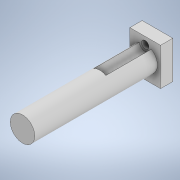
# Autodesk Inventor part: handle_vertical
Saved by Autodesk Inventor 2022.3 (Build 263350000, 350)
## iProperties
Created: 2022-06-10
Part Number: handle_vertical
Material: Generic
Document SubType Name: Modeling
Designer: Martijn
Density: 1 g/cm^3
Appearance: Default
Author: Martijn
Autodesk Inventor part; units mm, degrees
ref_plane "YZ Plane" through (0, 0, 0) normal (1, 0, 0) x (0, 1, 0)
ref_plane "XZ Plane" through (0, 0, 0) normal (0, 1, 0) x (-1, 0, 0)
ref_plane "XY Plane" through (0, 0, 0) normal (0, 0, 1) x (1, 0, 0)
sketch "Sketch1" plane through (0, 0, 0) normal (0, 0, 1) x (1, 0, 0)
  line L0 (0, 0) -> (25, 0)
  line L1 (25, 0) -> (25, 30.6)
  line L2 (25, 30.6) -> (0, 30.6)
  line L3 (0, 30.6) -> (0, 0)
  dimension "d0" = 25
  dimension "d1" = 30.6
  constraints: 8 end point, 2 parallel, 1 horizontal, 1 perpendicular
  measures "d0" distance of L0.start L0.end
  measures "d1" distance of L2.end L0.start
extrude "Extrusion1" add sketch "Sketch1" along normal blind 10
sketch "Sketch2" plane through (0, 0, 10) normal (0, 0, 1) x (1, 0, 0)
  circle A0 centre (12.5, 15.3) radius 10
  line L0 (25, 0) -> (25, 30.6) projected
  line L1 (0, 0) -> (25, 0) projected
  dimension "d4" = 12.5
  dimension "d6" = 20
  dimension "d19" = 15.3
  constraints: 1 centre point
  measures "d4" distance from line of L0 A0.centre
  measures "d6" diameter of A0
  measures "d19" distance from line of A0.centre L1
extrude "Extrusion2" add sketch "Sketch2" along normal blind 100
sketch "Sketch3" plane through (0, 0, 0) normal (0, 0, -1) x (-1, 0, 0)
  circle A0 centre (-12.5, 5.8) radius 3
  circle A1 centre (-12.5, 24.8) radius 3
  line L0 (0, 30.6) -> (0, 0) projected
  line L1 (0, 0) -> (-25, 0) projected
  point P0 (-12.5, 0)
  dimension "d9" = 6
  dimension "d10" = 6
  dimension "d11" = 12.5
  dimension "d12" = 12.5
  dimension "d13" = 19
  dimension "d14" = 5.8
  constraints: 2 centre point, 1 midpoint
  measures "d9" diameter of A0
  measures "d10" diameter of A1
  measures "d11" distance from line of L0 A0.centre
  measures "d12" distance from line of L0 A1.centre
  measures "d13" distance of A0.centre A1.centre
  measures "d14" distance of point (-12.5, 0) A0.centre
extrude "Extrusion3" cut sketch "Sketch3" against normal blind 20
sketch "Sketch4" plane through (0, 0, 10) normal (0, 0, 1) x (1, 0, 0)
  arc A0 (9.5003, 5.7605) -> (15.4997, 5.7605) centre (12.5, 5.8) ccw projected
  circle A1 centre (12.5, 5.8) radius 5
  arc A2 (15.4997, 24.8395) -> (9.5003, 24.8395) centre (12.5, 24.8) ccw projected
  circle A3 centre (12.5, 24.8) radius 5
  point P0 (0, 0)
  dimension "d17" = 10
  dimension "d18" = 10
  constraints: 2 centre point, 2 coincident
  measures "d17" diameter of A1
  measures "d18" diameter of A3
extrude "Extrusion4" cut sketch "Sketch4" along normal blind 37
body "Solid1"
